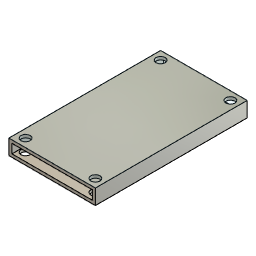
Cellule chauffante v3 (Autodesk Fusion 360 design; units mm, degrees)
Autodesk Fusion 360 part; units mm, degrees
sketch "Esquisse1" plane through (0, 0, 0) normal (0, 1, 0) x (1, 0, 0)
  line L0 (0, 0) -> (28.5, 0)
  line L1 (28.5, 0) -> (28.5, -50)
  line L2 (28.5, -50) -> (0, -50)
  line L3 (0, -50) -> (0, 0)
  circle A0 centre (2.75, -2.75) radius 1.5
  circle A1 centre (25.75, -2.75) radius 1.5
  circle A2 centre (2.75, -47.25) radius 1.5
  circle A3 centre (25.75, -47.25) radius 1.5
  dimension "d1" = 28.5
  dimension "d2" = 50
  dimension "d3" = 3
  dimension "d4" = 3
  dimension "d5" = 3
  dimension "d6" = 3
  dimension "d7" = 2.75
  dimension "d8" = 2.75
  dimension "d9" = 2.75
  dimension "d10" = 2.75
  dimension "d11" = 2.75
  dimension "d12" = 2.75
  dimension "d13" = 2.75
  dimension "d14" = 2.75
  constraint horizontal L0
  constraint vertical L1
  constraint horizontal L2
  constraint vertical L3
  constraint coincident L0.start L3.end
  measures "d1" distance of L0.start L0.end
  measures "d2" distance of L0.end L1.end
  measures "d3" diameter of A2
  measures "d4" diameter of A3
  measures "d5" diameter of A1
  measures "d6" diameter of A0
  measures "d7" distance of L0 A0.centre
  measures "d8" distance of L3 A0.centre
  measures "d9" distance of L0 A1.centre
  measures "d10" distance of L1 A1.centre
  measures "d11" distance of L3 A2.centre
  measures "d12" distance of L2 A2.centre
  measures "d13" distance of L2 A3.centre
  measures "d14" distance of L1 A3.centre
extrude "Extrusion1" add sketch "Esquisse1" along normal blind 5
sketch "Esquisse2" plane through (0, 0, 0) normal (0, 0, -1) x (-1, 0, 0)
  line L0 (-28.5, 0) -> (0, 0)
  line L1 (0, 0) -> (0, 5)
  line L2 (0, 5) -> (-28.5, 5)
  line L3 (-28.5, 5) -> (-28.5, 0)
  line L4 (-27.5, 4) -> (-1, 4)
  line L5 (-1, 4) -> (-1, 1)
  line L6 (-1, 1) -> (-27.5, 1)
  line L7 (-27.5, 1) -> (-27.5, 4)
  dimension "d17" = 1
  dimension "d18" = 1
  dimension "d19" = 1
  dimension "d20" = 1
  constraint horizontal L4
  constraint vertical L5
  constraint horizontal L6
  constraint vertical L7
  measures "d17" distance of L2 L4
  measures "d18" distance of L3 L7
  measures "d19" distance of L0 L6
  measures "d20" distance of L1 L5
extrude "Extrusion2" cut sketch "Esquisse2" against normal blind 71 contours L4 L5 L6 L7
sketch "Esquisse3" plane through (0, 5, 0) normal (0, 1, 0) x (-1, 0, 0)
  circle A0 centre (-2.75, 2.75) radius 1.5
  circle A1 centre (-2.75, 47.25) radius 1.5
  circle A2 centre (-25.75, 2.75) radius 1.5
  circle A3 centre (-25.75, 47.25) radius 1.5
  line L0 (0, 50) -> (-28.5, 50)
  line L1 (-28.5, 50) -> (-28.5, 0)
  line L2 (-28.5, 0) -> (0, 0)
  line L3 (0, 0) -> (0, 50)
